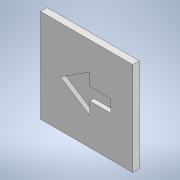
# Autodesk Inventor part: Part2
Saved by Autodesk Inventor 2022 (Build 260153000, 153)
## iProperties
Created: 2022-06-06
Part Number: Part2
Material: Generic
Document SubType Name: Modeling
Designer: tecware
Density: 1 g/cm^3
Appearance: Default
Author: tecware
## iProperties of the stored document Part2_3DPrint.ipt
Created: 2022-06-06
Part Number: Part2_3DPrint
Material: Generic
Document SubType Name: Modeling
Designer: tecware
Density: 1 g/cm^3
Appearance: Default
Author: tecware
Autodesk Inventor part; units mm, degrees
ref_plane "YZ Plane" through (0, 0, 0) normal (1, 0, 0) x (0, 1, 0)
ref_plane "XZ Plane" through (0, 0, 0) normal (0, 1, 0) x (-1, 0, 0)
ref_plane "XY Plane" through (0, 0, 0) normal (0, 0, 1) x (1, 0, 0)
sketch "Sketch1" plane through (0, 0, 0) normal (1, 0, 0) x (0, 1, 0)
  line L0 (11.1495, -7.3) -> (-11.1495, -7.3)
  line L1 (-11.1495, -7.3) -> (-11.1495, -5.7)
  line L2 (-11.1495, -5.7) -> (11.1495, -5.7)
  line L3 (11.1495, -5.7) -> (11.1495, -7.3)
  line L4 (11.1495, -7.3) -> (-11.1495, -5.7) construction
  line L5 (-11.1495, -7.3) -> (11.1495, -5.7) construction
  point P0 (0, 0)
  point P1 (0, -6.5)
  dimension "d1" = 22.299
  dimension "d2" = 1.6
  constraints: 12 end point, 2 midpoint
  measures "d1" distance of L1.end L2.end
  measures "d2" distance of L0.end L1.end
extrude "Extrusion1" add sketch "Sketch1" along normal mid plane 22
sketch "Sketch2" plane through (-11, -11.1495, -5.7) normal (0, 0, 1) x (1, 0, 0)
  line L0 (11.7587, 9.6495) -> (16.7587, 9.6495)
  line L1 (16.7587, 9.6495) -> (16.7587, 12.6495)
  line L2 (16.7587, 12.6495) -> (11.7587, 12.6495)
  line L3 (11.7587, 15.6495) -> (11.7587, 6.6495)
  line L4 (11.7587, 11.1495) -> (4.7587, 11.1495) construction
  line L5 (4.7587, 11.1495) -> (11.7587, 6.6495)
  line L6 (4.7587, 11.1495) -> (11.7587, 15.6495)
  line L7 (16.7587, 11.1495) -> (18.5587, 11.1495) construction
  line L8 (0, 22.299) -> (0, 0) projected
  point P0 (11.7587, 11.1495)
  point P1 (11.7587, 12.6495)
  dimension "d6" = 3
  dimension "d9" = 9
  dimension "d10" = 7
  dimension "d11" = 5
  dimension "d14" = 5
  constraints: 16 end point, 2 midpoint, 1 collinear, 1 parallel
  measures "d6" distance of L0.end L1.end
  measures "d9" distance of L3.start L3.end
  measures "d10" distance of L4.start L4.end
  measures "d11" distance between parallel lines of L1 L3
  measures "d14" distance of L0.start L0.end
extrude "Extrusion2" cut sketch "Sketch2" against normal blind 1
equation "\"d14\" = d11"
body "Solid1"
